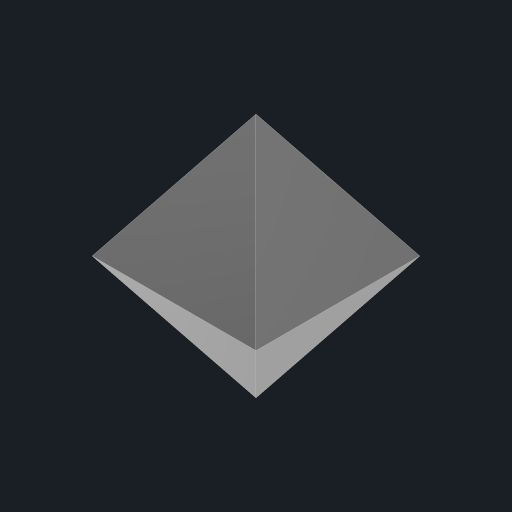
# Autodesk Inventor part: Dice, Simplified
Saved by Autodesk Inventor 2024.2 (Build 282272000, 272)
## iProperties
Created: 2024-11-22
Part Number: Dice, Simplified
Material: PVC-Piping
Document SubType Name: Modeling
Designer: Bryan
Mass: 5873.12 g
Surface Area: 1488.74 cm^2
Volume: 4195.09 cm^3
Density: 1.4 g/cm^3
Appearance: Smooth - Black
Author: Bryan
Autodesk Inventor part; units mm, degrees
ref_plane "YZ Plane" through (0, 0, 0) normal (1, 0, 0) x (0, 1, 0)
ref_plane "XZ Plane" through (0, 0, 0) normal (0, 1, 0) x (-1, 0, 0)
ref_plane "XY Plane" through (0, 0, 0) normal (0, 0, 1) x (1, 0, 0)
sketch "Sketch1" plane through (0, 0, 0) normal (0, 1, 0) x (-1, 0, 0)
  line L0 (-101.6, -101.6) -> (101.6, -101.6)
  line L1 (101.6, -101.6) -> (101.6, 101.6)
  line L2 (101.6, 101.6) -> (-101.6, 101.6)
  line L3 (-101.6, 101.6) -> (-101.6, -101.6)
  line L4 (-101.6, -101.6) -> (101.6, 101.6) construction
  line L5 (101.6, -101.6) -> (-101.6, 101.6) construction
  point P0 (0, 0)
  dimension "d0" = 203.2
  dimension "d1" = 203.2
  constraints: 12 end point, 2 midpoint, 2 parallel, 1 horizontal, 1 perpendicular
  measures "d0" distance of L2.end L1.end
  measures "d1" distance of L1.end L0.end
extrude "Extrusion1" add sketch "Sketch1" along normal mid plane 304.8
sketch "Sketch2" plane through (101.6, -152.4, -101.6) normal (1, 0, 0) x (0, 0, -1)
  line L0 (0, 304.8) -> (-203.2, 304.8) projected
  line L1 (-101.6, 304.8) -> (-203.2, 152.4)
  line L2 (-203.2, 0) -> (-203.2, 304.8) projected
  line L3 (-203.2, 152.4) -> (-101.6, 0)
  line L4 (0, 0) -> (-203.2, 0) projected
  line L5 (-101.6, 0) -> (0, 152.4)
  line L6 (0, 0) -> (0, 304.8) projected
  line L7 (-101.6, 304.8) -> (0, 152.4)
  point P0 (-101.6, 152.4)
  constraints: 8 end point, 4 midpoint
extrude "Extrusion2" cut sketch "Sketch2" against normal blind 304.8 contours L6 L7 L0 | L1 L2 L0 | L6 L4 L5 | L3 L4 L2
sketch "Sketch3" plane through (0, 0, 0) normal (0, 0, 1) x (1, 0, 0)
  line L0 (-101.6, 152.4) -> (101.6, 152.4) projected
  line L1 (0, 152.4) -> (-101.6, 0)
  line L2 (-101.6, 0) -> (0, -152.4)
  line L3 (-101.6, -152.4) -> (101.6, -152.4) projected
  line L4 (101.6, 0) -> (101.6, -152.4) projected
  line L5 (101.6, 0) -> (0, 152.4)
  line L6 (101.6, 0) -> (0, -152.4)
  line L7 (-101.6, 0) -> (-101.6, 152.4) projected
  line L8 (-101.6, 0) -> (101.6, 0) projected
  line L9 (101.6, 152.4) -> (101.6, 0) projected
  line L10 (-101.6, 152.4) -> (101.6, 152.4) projected
  line L11 (-101.6, -152.4) -> (-101.6, 0) projected
  line L12 (-101.6, -152.4) -> (101.6, -152.4) projected
  line L13 (101.6, 0) -> (101.6, -152.4) projected
  line L14 (-101.6, 0) -> (101.6, 0) projected
  point P0 (0, 0)
  constraints: 8 end point, 2 midpoint, 2 parallel
extrude "Extrusion3" cut sketch "Sketch3" along normal through all both and the other way through all contours L0 L1 L7 | L0 L9 L5 | L2 L3 L11 | L4 L3 L6
body "Solid1"
